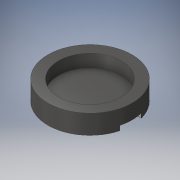
# Autodesk Inventor part: Lower Power
Saved by Autodesk Inventor 2016 (Build 200138000, 138)
## iProperties
Created: 2018-04-23
Part Number: Lower Power
Material: Generic
Document SubType Name: Modeling
Designer: student
Density: 1 g/cm^3
Appearance: Default
Author: student
Autodesk Inventor part; units mm, degrees
ref_plane "YZ Plane" through (0, 0, 0) normal (1, 0, 0) x (0, 1, 0)
ref_plane "XZ Plane" through (0, 0, 0) normal (0, 1, 0) x (-1, 0, 0)
ref_plane "XY Plane" through (0, 0, 0) normal (0, 0, 1) x (1, 0, 0)
sketch "Sketch1" plane through (0, 0, 0) normal (0, 1, 0) x (-1, 0, 0)
  circle A0 centre (0, 0) radius 18.542 construction
  circle A1 centre (0, 0) radius 24.892
  dimension "d0" = 37.084
  dimension "d1" = 6.35
  constraints: 2 centre point, 2 coincident
  measures "d0" diameter of A0
  measures "d1" radial gap between concentric circles of A1 A0
extrude "Extrusion1" add sketch "Sketch1" along normal blind 11.43
sketch "Sketch2" plane through (0, 11.43, 0) normal (0, 1, 0) x (1, 0, 0)
  circle A0 centre (0, 0) radius 18.669
  dimension "d4" = 37.338
  constraints: 1 centre point, 1 coincident
  measures "d4" diameter of A0
extrude "Extrusion2" cut sketch "Sketch2" against normal blind 7.62
sketch "Sketch3" plane through (0, 0, 0) normal (0, -1, 0) x (1, 0, 0)
  circle A0 centre (0, 0) radius 22.1615
  circle A1 centre (0, 0) radius 9.779
  dimension "d7" = 44.323
  dimension "d10" = 19.558
  constraints: 2 centre point, 2 coincident
  measures "d7" diameter of A0
  measures "d10" diameter of A1
extrude "Extrusion4" cut sketch "Sketch3" against normal blind 2.7178
sketch "Sketch4" plane through (0, 0, 0) normal (0, -1, 0) x (1, 0, 0)
  line L0 (31.242, -6.35) -> (18.542, -6.35)
  line L1 (18.542, -6.35) -> (18.542, 6.35)
  line L2 (18.542, 6.35) -> (31.242, 6.35)
  line L3 (31.242, 6.35) -> (31.242, -6.35)
  circle A0 centre (0, 0) radius 24.892 projected
  line L4 (31.242, -6.35) -> (18.542, 6.35) construction
  line L5 (18.542, -6.35) -> (31.242, 6.35) construction
  point P0 (24.892, 0)
  dimension "d13" = 12.7
  dimension "d14" = 12.7
  constraints: 12 end point, 2 midpoint, 2 parallel, 1 horizontal, 1 horizontal alignment, 1 perpendicular, 1 other
  measures "d13" distance of L1.end L2.end
  measures "d14" distance of L0.end L1.end
extrude "Extrusion5" cut sketch "Sketch4" against normal up to surface (2.7178 mm away) contours L0 A0 L2 L3 | L0 L1 L2 A0 picked at (20.6587, 0)
body "Solid1"
